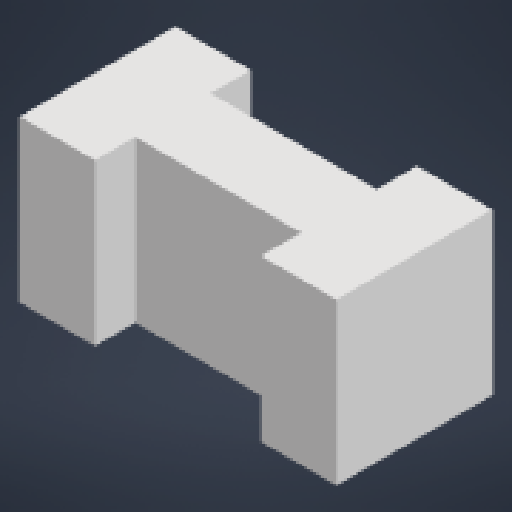
# Autodesk Inventor part: outerdisk_pin
Saved by Autodesk Inventor 2026 (Build 300175050, 175E)
## iProperties
Created: 2026-04-01
Part Number: outerdisk_pin
Material: Generic
Document SubType Name: Modeling
Designer: sniel
Density: 1 g/cm^3
Appearance: Default
Author: sniel
Autodesk Inventor part; units mm, degrees
ref_plane "YZ Plane" through (0, 0, 0) normal (1, 0, 0) x (0, 1, 0)
ref_plane "XZ Plane" through (0, 0, 0) normal (0, 1, 0) x (-1, 0, 0)
ref_plane "XY Plane" through (0, 0, 0) normal (0, 0, 1) x (1, 0, 0)
sketch "Sketch1" plane through (0, 0, 0) normal (0, 1, 0) x (-1, 0, 0)
  line L0 (0, -2.5) -> (0, 2.5)
  line L1 (5, 2.5) -> (0, 2.5)
  line L2 (5, 5) -> (5, 2.5)
  line L3 (10, 5) -> (5, 5)
  line L4 (10, -5) -> (10, 5)
  line L5 (5, -5) -> (10, -5)
  line L6 (5, -2.5) -> (5, -5)
  line L7 (0, -2.5) -> (5, -2.5)
  line L8 (0, 0) -> (10, 0)
  line L9 (0, 8) -> (0, -11)
  line L10 (-5, 2.5) -> (0, 2.5)
  line L11 (-5, 5) -> (-5, 2.5)
  line L12 (-10, 5) -> (-5, 5)
  line L13 (-10, -5) -> (-10, 5)
  line L14 (-5, -5) -> (-10, -5)
  line L15 (-5, -2.5) -> (-5, -5)
  line L16 (0, -2.5) -> (-5, -2.5)
  line L17 (0, 0) -> (-10, 0)
  line L18 (-10, 5) -> (-9.85, 5)
  line L19 (-9.85, 5) -> (-9.85, 4.85)
  line L20 (-9.85, 4.85) -> (-10, 4.85)
  line L21 (-10, 4.85) -> (-10, 5)
  line L22 (-10, -5) -> (-9.85, -5)
  line L23 (-9.85, -5) -> (-9.85, -4.85)
  line L24 (-9.85, -4.85) -> (-10, -4.85)
  line L25 (-10, -4.85) -> (-10, -5)
  line L26 (-5, 5) -> (-5.15, 5)
  line L27 (-5.15, 5) -> (-5.15, 4.85)
  line L28 (-5.15, 4.85) -> (-5, 4.85)
  line L29 (-5, 4.85) -> (-5, 5)
  line L30 (-5, -5) -> (-5.15, -5)
  line L31 (-5.15, -5) -> (-5.15, -4.85)
  line L32 (-5.15, -4.85) -> (-5, -4.85)
  line L33 (-5, -4.85) -> (-5, -5)
  line L34 (-5, -2.5) -> (-5.15, -2.5)
  line L35 (-5.15, -2.5) -> (-5.15, -2.35)
  line L36 (-5.15, -2.35) -> (-5, -2.35)
  line L37 (-5, -2.35) -> (-5, -2.5)
  line L38 (-5, 2.5) -> (-5.15, 2.5)
  line L39 (-5.15, 2.5) -> (-5.15, 2.35)
  line L40 (-5.15, 2.35) -> (-5, 2.35)
  line L41 (-5, 2.35) -> (-5, 2.5)
  line L42 (5, 2.5) -> (5.15, 2.5)
  line L43 (5.15, 2.5) -> (5.15, 2.35)
  line L44 (5.15, 2.35) -> (5, 2.35)
  line L45 (5, 2.35) -> (5, 2.5)
  line L46 (5, 5) -> (5.15, 5)
  line L47 (5.15, 5) -> (5.15, 4.85)
  line L48 (5.15, 4.85) -> (5, 4.85)
  line L49 (5, 4.85) -> (5, 5)
  line L50 (10, 5) -> (9.85, 5)
  line L51 (9.85, 5) -> (9.85, 4.85)
  line L52 (9.85, 4.85) -> (10, 4.85)
  line L53 (10, 4.85) -> (10, 5)
  line L54 (10, -5) -> (9.85, -5)
  line L55 (9.85, -5) -> (9.85, -4.85)
  line L56 (9.85, -4.85) -> (10, -4.85)
  line L57 (10, -4.85) -> (10, -5)
  line L58 (5, -5) -> (5.15, -5)
  line L59 (5.15, -5) -> (5.15, -4.85)
  line L60 (5.15, -4.85) -> (5, -4.85)
  line L61 (5, -4.85) -> (5, -5)
  line L62 (5, -2.5) -> (5.15, -2.5)
  line L63 (5.15, -2.5) -> (5.15, -2.35)
  line L64 (5.15, -2.35) -> (5, -2.35)
  line L65 (5, -2.35) -> (5, -2.5)
  line L66 (5.15, 4.85) -> (9.85, 4.85)
  line L67 (9.85, 4.85) -> (9.85, -4.85)
  line L68 (9.85, -4.85) -> (5.15, -4.85)
  line L69 (5.15, -4.85) -> (5.15, 4.85)
  line L70 (-5.15, 4.85) -> (-9.85, 4.85)
  line L71 (-9.85, 4.85) -> (-9.85, -4.85)
  line L72 (-9.85, -4.85) -> (-5.15, -4.85)
  line L73 (-5.15, -4.85) -> (-5.15, 4.85)
  line L74 (-5.15, 2.35) -> (5.15, 2.35)
  line L75 (5.15, 2.35) -> (5.15, -2.35)
  line L76 (5.15, -2.35) -> (-5.15, -2.35)
  line L77 (-5.15, -2.35) -> (-5.15, 2.35)
  dimension "d0" = 0.15
  dimension "d1" = 0.15
  dimension "d2" = 0.15
  dimension "d3" = 0.15
  dimension "d4" = 0.15
  dimension "d5" = 0.15
  dimension "d6" = 0.15
  dimension "d7" = 0.15
  dimension "d8" = 0.15
  dimension "d9" = 0.15
  dimension "d10" = 0.15
  dimension "d11" = 0.15
  dimension "d12" = 0.15
  dimension "d13" = 0.15
  dimension "d14" = 0.15
  dimension "d15" = 0.15
  dimension "d16" = 0.15
  dimension "d17" = 0.15
  dimension "d18" = 0.15
  dimension "d19" = 0.15
  dimension "d20" = 0.15
  dimension "d21" = 0.15
  dimension "d22" = 0.15
  dimension "d23" = 0.15
  constraints: 156 end point, 30 parallel, 15 horizontal, 15 perpendicular, 7 symmetric about line, 2 midpoint
  measures "d0" distance of L19.end L20.end
  measures "d1" distance of L18.end L19.end
  measures "d2" distance of L24.end L23.end
  measures "d3" distance of L23.end L22.end
  measures "d4" distance of L28.end L27.end
  measures "d5" distance of L27.end L26.end
  measures "d6" distance of L31.end L32.end
  measures "d7" distance of L30.end L31.end
  measures "d8" distance of L35.end L36.end
  measures "d9" distance of L34.end L35.end
  measures "d10" distance of L40.end L39.end
  measures "d11" distance of L39.end L38.end
  measures "d12" distance of L43.end L44.end
  measures "d13" distance of L42.end L43.end
  measures "d14" distance of L47.end L48.end
  measures "d15" distance of L46.end L47.end
  measures "d16" distance of L52.end L51.end
  measures "d17" distance of L51.end L50.end
  measures "d18" distance of L55.end L56.end
  measures "d19" distance of L54.end L55.end
  measures "d20" distance of L60.end L59.end
  measures "d21" distance of L59.end L58.end
  measures "d22" distance of L64.end L63.end
  measures "d23" distance of L63.end L62.end
extrude "Extrusion1" add sketch "Sketch1" along normal blind 5 contours L76 L36 L73 L17 L0 | L0 L8 L69 L64 L76 | L17 L73 L40 L74 L0 | L0 L74 L44 L69 L8 | L63 L69 L8 L67 L68 | L73 L72 L71 L17 L35 | L69 L43 L66 L67 L8 | L17 L71 L70 L73 L39
body "Solid1"
